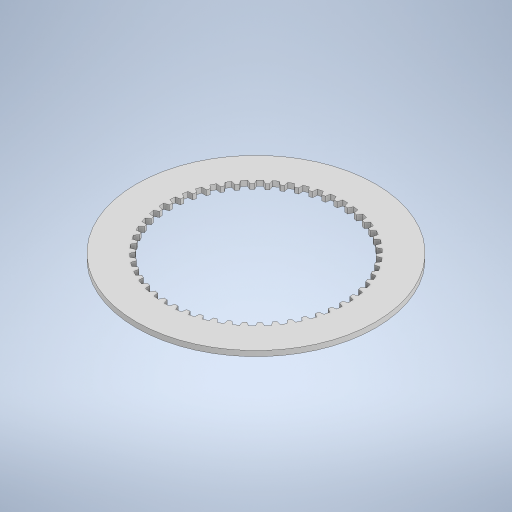
# Autodesk Inventor part: AP-1-01-ring50tooth
Saved by Autodesk Inventor 2023 (Build 270158000, 158)
## iProperties
Created: 2023-06-27
Part Number: AP-1-01-ring50tooth
Material: Generic
Document SubType Name: Modeling
Designer: t205b
Density: 1 g/cm^3
Appearance: Default
Author: t205b
Autodesk Inventor part; units mm, degrees
ref_plane "YZ Plane" through (0, 0, 0) normal (1, 0, 0) x (0, 1, 0)
ref_plane "XZ Plane" through (0, 0, 0) normal (0, 1, 0) x (-1, 0, 0)
ref_plane "XY Plane" through (0, 0, 0) normal (0, 0, 1) x (1, 0, 0)
sketch "Sketch1" plane through (0, 0, 0) normal (0, 1, 0) x (-1, 0, 0)
  circle A0 centre (0, 0) radius 113.75
  circle A1 centre (0, 0) radius 85
  line L0 (-84.947, -3) -> (-81, -1.5)
  line L1 (-81, -1.5) -> (-81, 1.5)
  line L2 (-81, 1.5) -> (-84.947, 3)
  line L3 (-83.9012, -13.623) -> (-80.1733, -11.6402)
  line L4 (-80.1733, -11.6402) -> (-80.5493, -8.6638)
  line L5 (-80.5493, -8.6638) -> (-84.6532, -7.6703)
  line L6 (-81.5322, -24.0312) -> (-78.0822, -21.5968)
  line L7 (-78.0822, -21.5968) -> (-78.8283, -18.691)
  line L8 (-78.8283, -18.691) -> (-83.0243, -18.2197)
  line L9 (-77.8774, -34.0604) -> (-74.7597, -31.2128)
  line L10 (-74.7597, -31.2128) -> (-75.8641, -28.4234)
  line L11 (-75.8641, -28.4234) -> (-80.0861, -28.4818)
  line L12 (-72.9944, -43.5525) -> (-70.2582, -40.3365)
  line L13 (-70.2582, -40.3365) -> (-71.7035, -37.7076)
  line L14 (-71.7035, -37.7076) -> (-75.8849, -38.2946)
  line L15 (-66.9602, -52.3577) -> (-64.6487, -48.8241)
  line L16 (-64.6487, -48.8241) -> (-66.4121, -46.3971)
  line L17 (-66.4121, -46.3971) -> (-70.487, -47.5036)
  line L18 (-59.8701, -60.3372) -> (-58.0196, -56.5418)
  line L19 (-58.0196, -56.5418) -> (-60.0733, -54.3549)
  line L20 (-60.0733, -54.3549) -> (-63.9774, -55.9633)
  line L21 (-51.8357, -67.3651) -> (-50.4756, -63.3677)
  line L22 (-50.4756, -63.3677) -> (-52.7871, -61.4554)
  line L23 (-52.7871, -61.4554) -> (-56.4588, -63.5405)
  line L24 (-42.9839, -73.3306) -> (-42.1355, -69.1943)
  line L25 (-42.1355, -69.1943) -> (-44.6685, -67.5868)
  line L26 (-44.6685, -67.5868) -> (-48.0499, -70.1157)
  line L27 (-33.4542, -78.1397) -> (-33.1309, -73.9297)
  line L28 (-33.1309, -73.9297) -> (-35.8454, -72.6523)
  line L29 (-35.8454, -72.6523) -> (-38.8832, -75.585)
  line L30 (-23.3969, -81.7165) -> (-23.6038, -77.4991)
  line L31 (-23.6038, -77.4991) -> (-26.457, -76.5721)
  line L32 (-26.457, -76.5721) -> (-29.1032, -79.8624)
  line L33 (-12.9706, -84.0045) -> (-13.7045, -79.8463)
  line L34 (-13.7045, -79.8463) -> (-16.6513, -79.2842)
  line L35 (-16.6513, -79.2842) -> (-18.8644, -82.8803)
  line L36 (-2.3398, -84.9678) -> (-3.589, -80.9344)
  line L37 (-3.589, -80.9344) -> (-6.5831, -80.746)
  line L38 (-6.5831, -80.746) -> (-8.3279, -84.591)
  line L39 (8.3279, -84.591) -> (6.5831, -80.746)
  line L40 (6.5831, -80.746) -> (3.589, -80.9344)
  line L41 (3.589, -80.9344) -> (2.3398, -84.9678)
  line L42 (18.8644, -82.8803) -> (16.6513, -79.2842)
  line L43 (16.6513, -79.2842) -> (13.7045, -79.8463)
  line L44 (13.7045, -79.8463) -> (12.9706, -84.0045)
  line L45 (29.1032, -79.8624) -> (26.457, -76.5721)
  line L46 (26.457, -76.5721) -> (23.6038, -77.4991)
  line L47 (23.6038, -77.4991) -> (23.3969, -81.7165)
  line L48 (38.8832, -75.585) -> (35.8454, -72.6523)
  line L49 (35.8454, -72.6523) -> (33.1309, -73.9297)
  line L50 (33.1309, -73.9297) -> (33.4542, -78.1397)
  line L51 (48.0499, -70.1157) -> (44.6685, -67.5868)
  line L52 (44.6685, -67.5868) -> (42.1355, -69.1943)
  line L53 (42.1355, -69.1943) -> (42.9839, -73.3306)
  line L54 (56.4588, -63.5405) -> (52.7871, -61.4554)
  line L55 (52.7871, -61.4554) -> (50.4756, -63.3677)
  line L56 (50.4756, -63.3677) -> (51.8357, -67.3651)
  line L57 (63.9774, -55.9633) -> (60.0733, -54.3549)
  line L58 (60.0733, -54.3549) -> (58.0196, -56.5418)
  line L59 (58.0196, -56.5418) -> (59.8701, -60.3372)
  line L60 (70.487, -47.5036) -> (66.4121, -46.3971)
  line L61 (66.4121, -46.3971) -> (64.6487, -48.8241)
  line L62 (64.6487, -48.8241) -> (66.9602, -52.3577)
  line L63 (75.8849, -38.2946) -> (71.7035, -37.7076)
  line L64 (71.7035, -37.7076) -> (70.2582, -40.3365)
  line L65 (70.2582, -40.3365) -> (72.9944, -43.5525)
  line L66 (80.0861, -28.4818) -> (75.8641, -28.4234)
  line L67 (75.8641, -28.4234) -> (74.7597, -31.2128)
  line L68 (74.7597, -31.2128) -> (77.8774, -34.0604)
  line L69 (83.0243, -18.2197) -> (78.8283, -18.691)
  line L70 (78.8283, -18.691) -> (78.0822, -21.5968)
  line L71 (78.0822, -21.5968) -> (81.5322, -24.0312)
  line L72 (84.6532, -7.6703) -> (80.5493, -8.6638)
  line L73 (80.5493, -8.6638) -> (80.1733, -11.6402)
  line L74 (80.1733, -11.6402) -> (83.9012, -13.623)
  line L75 (84.947, 3) -> (81, 1.5)
  line L76 (81, 1.5) -> (81, -1.5)
  line L77 (81, -1.5) -> (84.947, -3)
  line L78 (83.9012, 13.623) -> (80.1733, 11.6402)
  line L79 (80.1733, 11.6402) -> (80.5493, 8.6638)
  line L80 (80.5493, 8.6638) -> (84.6532, 7.6703)
  line L81 (81.5322, 24.0312) -> (78.0822, 21.5968)
  line L82 (78.0822, 21.5968) -> (78.8283, 18.691)
  line L83 (78.8283, 18.691) -> (83.0243, 18.2197)
  line L84 (77.8774, 34.0604) -> (74.7597, 31.2128)
  line L85 (74.7597, 31.2128) -> (75.8641, 28.4234)
  line L86 (75.8641, 28.4234) -> (80.0861, 28.4818)
  line L87 (72.9944, 43.5525) -> (70.2582, 40.3365)
  line L88 (70.2582, 40.3365) -> (71.7035, 37.7076)
  line L89 (71.7035, 37.7076) -> (75.8849, 38.2946)
  line L90 (66.9602, 52.3577) -> (64.6487, 48.8241)
  line L91 (64.6487, 48.8241) -> (66.4121, 46.3971)
  line L92 (66.4121, 46.3971) -> (70.487, 47.5036)
  line L93 (59.8701, 60.3372) -> (58.0196, 56.5418)
  line L94 (58.0196, 56.5418) -> (60.0733, 54.3549)
  line L95 (60.0733, 54.3549) -> (63.9774, 55.9633)
  line L96 (51.8357, 67.3651) -> (50.4756, 63.3677)
  line L97 (50.4756, 63.3677) -> (52.7871, 61.4554)
  line L98 (52.7871, 61.4554) -> (56.4588, 63.5405)
  line L99 (42.9839, 73.3306) -> (42.1355, 69.1943)
  line L100 (42.1355, 69.1943) -> (44.6685, 67.5868)
  line L101 (44.6685, 67.5868) -> (48.0499, 70.1157)
  line L102 (33.4542, 78.1397) -> (33.1309, 73.9297)
  line L103 (33.1309, 73.9297) -> (35.8454, 72.6523)
  line L104 (35.8454, 72.6523) -> (38.8832, 75.585)
  line L105 (23.3969, 81.7165) -> (23.6038, 77.4991)
  line L106 (23.6038, 77.4991) -> (26.457, 76.5721)
  line L107 (26.457, 76.5721) -> (29.1032, 79.8624)
  line L108 (12.9706, 84.0045) -> (13.7045, 79.8463)
  line L109 (13.7045, 79.8463) -> (16.6513, 79.2842)
  line L110 (16.6513, 79.2842) -> (18.8644, 82.8803)
  line L111 (2.3398, 84.9678) -> (3.589, 80.9344)
  line L112 (3.589, 80.9344) -> (6.5831, 80.746)
  line L113 (6.5831, 80.746) -> (8.3279, 84.591)
  line L114 (-8.3279, 84.591) -> (-6.5831, 80.746)
  line L115 (-6.5831, 80.746) -> (-3.589, 80.9344)
  line L116 (-3.589, 80.9344) -> (-2.3398, 84.9678)
  line L117 (-18.8644, 82.8803) -> (-16.6513, 79.2842)
  line L118 (-16.6513, 79.2842) -> (-13.7045, 79.8463)
  line L119 (-13.7045, 79.8463) -> (-12.9706, 84.0045)
  line L120 (-29.1032, 79.8624) -> (-26.457, 76.5721)
  line L121 (-26.457, 76.5721) -> (-23.6038, 77.4991)
  line L122 (-23.6038, 77.4991) -> (-23.3969, 81.7165)
  line L123 (-38.8832, 75.585) -> (-35.8454, 72.6523)
  line L124 (-35.8454, 72.6523) -> (-33.1309, 73.9297)
  line L125 (-33.1309, 73.9297) -> (-33.4542, 78.1397)
  line L126 (-48.0499, 70.1157) -> (-44.6685, 67.5868)
  line L127 (-44.6685, 67.5868) -> (-42.1355, 69.1943)
  line L128 (-42.1355, 69.1943) -> (-42.9839, 73.3306)
  line L129 (-56.4588, 63.5405) -> (-52.7871, 61.4554)
  line L130 (-52.7871, 61.4554) -> (-50.4756, 63.3677)
  line L131 (-50.4756, 63.3677) -> (-51.8357, 67.3651)
  line L132 (-63.9774, 55.9633) -> (-60.0733, 54.3549)
  line L133 (-60.0733, 54.3549) -> (-58.0196, 56.5418)
  line L134 (-58.0196, 56.5418) -> (-59.8701, 60.3372)
  line L135 (-70.487, 47.5036) -> (-66.4121, 46.3971)
  line L136 (-66.4121, 46.3971) -> (-64.6487, 48.8241)
  line L137 (-64.6487, 48.8241) -> (-66.9602, 52.3577)
  line L138 (-75.8849, 38.2946) -> (-71.7035, 37.7076)
  line L139 (-71.7035, 37.7076) -> (-70.2582, 40.3365)
  line L140 (-70.2582, 40.3365) -> (-72.9944, 43.5525)
  line L141 (-80.0861, 28.4818) -> (-75.8641, 28.4234)
  line L142 (-75.8641, 28.4234) -> (-74.7597, 31.2128)
  line L143 (-74.7597, 31.2128) -> (-77.8774, 34.0604)
  line L144 (-83.0243, 18.2197) -> (-78.8283, 18.691)
  line L145 (-78.8283, 18.691) -> (-78.0822, 21.5968)
  line L146 (-78.0822, 21.5968) -> (-81.5322, 24.0312)
  line L147 (-84.6532, 7.6703) -> (-80.5493, 8.6638)
  line L148 (-80.5493, 8.6638) -> (-80.1733, 11.6402)
  line L149 (-80.1733, 11.6402) -> (-83.9012, 13.623)
  dimension "d1" = 170
  dimension "d0" = 227.5
  dimension "d2" = 3
  dimension "d3" = 81
  dimension "d4" = 6
  dimension "d5" = 110.808
  dimension "d6" = 110.808
  dimension "d9" = 360
  constraints: 300 end point, 2 coincident, 1 centre point, 1 equal length, 1 vertical, 354 other
  measures "d0" diameter of A0
  measures "d2" distance of L0.end L1.end
  measures "d3" distance from line of L1 point (0, 0)
  measures "d4" distance of L2.end L0.start
  measures "d5" angle of L2 L1
  measures "d6" angle of L0 L1
extrude "Extrusion1" add sketch "Sketch1" along normal blind 5 contours A0 | A1 L77 L76 L75 | L80 L79 L78 A1 | A1 L74 L73 L72 | L83 L82 L81 A1 | A1 L71 L70 L69 | L86 L85 L84 A1 | A1 L68 L67 L66 | L89 L88 L87 A1 | A1 L65 L64 L63 | L92 L91 L90 A1 | A1 L62 L61 L60 | L95 L94 L93 A1 | A1 L59 L58 L57 | L98 L97 L96 A1 | A1 L56 L55 L54 | L101 L100 L99 A1 | A1 L53 L52 L51 | L104 L103 L102 A1 | A1 L50 L49 L48 | L107 L106 L105 A1 | A1 L47 L46 L45 | L110 L109 L108 A1 | A1 L44 L43 L42 | L113 L112 L111 A1 | A1 L41 L40 L39 | L116 L115 L114 A1 | A1 L38 L37 L36 | L119 L118 L117 A1 | A1 L35 L34 L33 | L122 L121 L120 A1 | A1 L32 L31 L30 | L125 L124 L123 A1 | A1 L29 L28 L27 | L128 L127 L126 A1 | A1 L26 L25 L24 | L131 L130 L129 A1 | A1 L23 L22 L21 | L134 L133 L132 A1 | A1 L20 L19 L18 | L137 L136 L135 A1 | A1 L17 L16 L15 | L140 L139 L138 A1 | A1 L14 L13 L12 | L143 L142 L141 A1 | A1 L11 L10 L9 | L146 L145 L144 A1 | A1 L8 L7 L6 | L149 L148 L147 A1 | A1 L5 L4 L3 | L2 L1 L0 A1
equation "\"d5\" = d6"
body "Solid1"
